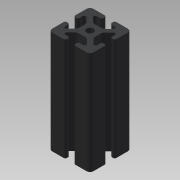
# Autodesk Inventor part: 40-4040-BLACK-FB
Saved by Autodesk Inventor 2013 (Build 170138000, 138)
## iProperties
Company: 80/20 Inc.
Created: 2014-04-23
Part Number: 40-4040-BLACK-FB
Material: Generic
Document SubType Name: Modeling
Designer: Ross Bowman
Density: 1 g/cm^3
Engineer: Ross Bowman
Catalog Web Link: 8020.net
Vendor: 80/20 Inc.
Material: 6105-T5 Aluminum
Author: Ross Bowman
Keywords: 80/20 , 8020 , T-Slot , Extrusion
Autodesk Inventor part; units mm, degrees
ref_plane "YZ Plane" through (0, 0, 0) normal (1, 0, 0) x (0, 1, 0)
ref_plane "XZ Plane" through (0, 0, 0) normal (0, 1, 0) x (-1, 0, 0)
ref_plane "XY Plane" through (0, 0, 0) normal (0, 0, 1) x (1, 0, 0)
sketch "Sketch1" plane through (0, 0, 0) normal (0, 0, 1) x (1, 0, 0)
  circle A0 centre (0, 0) radius 3.4
  arc A1 (-4.06, -17.0946) -> (-5.63, -15.5246) centre (-5.63, -17.0946) ccw
  line L0 (-5.63, -15.5246) -> (-8.715, -15.5246)
  arc A2 (-10.285, -13.9546) -> (-8.715, -15.5246) centre (-8.715, -13.9546) ccw
  line L1 (-10.285, -13.9546) -> (-10.285, -13.4925)
  arc A3 (-10.0624, -12.9551) -> (-10.285, -13.4925) centre (-9.525, -13.4925) ccw
  line L2 (-10.0624, -12.9551) -> (-6.2171, -9.1098)
  arc A4 (-2.7773, -7.685) -> (-6.2171, -9.1098) centre (-2.7773, -12.5496) ccw
  line L3 (-2.7773, -7.685) -> (2.7773, -7.685)
  arc A5 (6.2171, -9.1098) -> (2.7773, -7.685) centre (2.7773, -12.5496) ccw
  line L4 (6.2171, -9.1098) -> (10.0624, -12.9551)
  arc A6 (10.285, -13.4925) -> (10.0624, -12.9551) centre (9.525, -13.4925) ccw
  line L5 (10.285, -13.4925) -> (10.285, -13.9546)
  arc A7 (8.715, -15.5246) -> (10.285, -13.9546) centre (8.715, -13.9546) ccw
  line L6 (8.715, -15.5246) -> (5.63, -15.5246)
  arc A8 (5.63, -15.5246) -> (4.06, -17.0946) centre (5.63, -17.0946) ccw
  line L7 (4.06, -17.0946) -> (4.06, -18.43)
  arc A9 (4.06, -18.43) -> (5.63, -20) centre (5.63, -18.43) ccw
  line L8 (5.63, -20) -> (16.83, -20)
  arc A10 (16.83, -20) -> (20, -16.83) centre (16.83, -16.83) ccw
  line L9 (20, -16.83) -> (20, -5.63)
  arc A11 (20, -5.63) -> (18.43, -4.06) centre (18.43, -5.63) ccw
  line L10 (18.43, -4.06) -> (17.25, -4.06)
  arc A12 (17.25, -4.06) -> (15.68, -5.63) centre (17.25, -5.63) ccw
  line L11 (15.68, -5.63) -> (15.68, -8.7154)
  arc A13 (14.11, -10.2854) -> (15.68, -8.7154) centre (14.11, -8.7154) ccw
  line L12 (14.11, -10.2854) -> (13.6201, -10.2854)
  arc A14 (13.1637, -9.947) -> (13.6201, -10.2854) centre (13.8117, -9.55) ccw
  line L13 (13.1637, -9.947) -> (9.0762, -5.8595)
  arc A15 (7.685, -2.5008) -> (9.0762, -5.8595) centre (12.435, -2.5008) ccw
  line L14 (7.685, -2.5008) -> (7.685, 2.5008)
  arc A16 (9.0762, 5.8595) -> (7.685, 2.5008) centre (12.435, 2.5008) ccw
  line L15 (9.0762, 5.8595) -> (13.2795, 10.0628)
  arc A17 (13.8169, 10.2854) -> (13.2795, 10.0628) centre (13.8169, 9.5254) ccw
  line L16 (13.8169, 10.2854) -> (14.11, 10.2854)
  arc A18 (15.68, 8.7154) -> (14.11, 10.2854) centre (14.11, 8.7154) ccw
  line L17 (15.68, 8.7154) -> (15.68, 5.63)
  arc A19 (15.68, 5.63) -> (17.25, 4.06) centre (17.25, 5.63) ccw
  line L18 (17.25, 4.06) -> (18.43, 4.06)
  arc A20 (18.43, 4.06) -> (20, 5.63) centre (18.43, 5.63) ccw
  line L19 (20, 5.63) -> (20, 16.83)
  arc A21 (20, 16.83) -> (16.83, 20) centre (16.83, 16.83) ccw
  line L20 (16.83, 20) -> (5.63, 20)
  arc A22 (5.63, 20) -> (4.06, 18.43) centre (5.63, 18.43) ccw
  line L21 (4.06, 18.43) -> (4.06, 17.0946)
  arc A23 (4.06, 17.0946) -> (5.63, 15.5246) centre (5.63, 17.0946) ccw
  line L22 (5.63, 15.5246) -> (8.715, 15.5246)
  arc A24 (10.285, 13.9546) -> (8.715, 15.5246) centre (8.715, 13.9546) ccw
  line L23 (10.285, 13.9546) -> (10.285, 13.4925)
  arc A25 (10.0624, 12.9551) -> (10.285, 13.4925) centre (9.525, 13.4925) ccw
  line L24 (10.0624, 12.9551) -> (6.2171, 9.1098)
  arc A26 (2.7773, 7.685) -> (6.2171, 9.1098) centre (2.7773, 12.5496) ccw
  line L25 (2.7773, 7.685) -> (-2.7773, 7.685)
  arc A27 (-6.2171, 9.1098) -> (-2.7773, 7.685) centre (-2.7773, 12.5496) ccw
  line L26 (-6.2171, 9.1098) -> (-10.0624, 12.9551)
  arc A28 (-10.285, 13.4925) -> (-10.0624, 12.9551) centre (-9.525, 13.4925) ccw
  line L27 (-10.285, 13.4925) -> (-10.285, 13.9546)
  arc A29 (-8.715, 15.5246) -> (-10.285, 13.9546) centre (-8.715, 13.9546) ccw
  line L28 (-8.715, 15.5246) -> (-5.63, 15.5246)
  arc A30 (-5.63, 15.5246) -> (-4.06, 17.0946) centre (-5.63, 17.0946) ccw
  line L29 (-4.06, 17.0946) -> (-4.06, 18.43)
  arc A31 (-4.06, 18.43) -> (-5.63, 20) centre (-5.63, 18.43) ccw
  line L30 (-5.63, 20) -> (-16.83, 20)
  arc A32 (-16.83, 20) -> (-20, 16.83) centre (-16.83, 16.83) ccw
  line L31 (-20, 16.83) -> (-20, 5.573)
  arc A33 (-20, 5.573) -> (-18.43, 4.003) centre (-18.43, 5.573) ccw
  line L32 (-18.43, 4.003) -> (-17.25, 4.003)
  arc A34 (-17.25, 4.003) -> (-15.68, 5.573) centre (-17.25, 5.573) ccw
  line L33 (-15.68, 5.573) -> (-15.68, 8.4757)
  arc A35 (-14.0552, 10.0447) -> (-15.68, 8.4757) centre (-14.11, 8.4757) ccw
  line L34 (-14.0552, 10.0447) -> (-13.7199, 10.033)
  arc A36 (-13.0405, 9.8238) -> (-13.7199, 10.033) centre (-13.5779, 9.2864) ccw
  line L35 (-13.0405, 9.8238) -> (-9.0762, 5.8595)
  arc A37 (-7.685, 2.5008) -> (-9.0762, 5.8595) centre (-12.435, 2.5008) ccw
  line L36 (-7.685, 2.5008) -> (-7.685, -2.5008)
  arc A38 (-9.0762, -5.8595) -> (-7.685, -2.5008) centre (-12.435, -2.5008) ccw
  line L37 (-9.0762, -5.8595) -> (-13.2795, -10.0628)
  arc A39 (-13.8169, -10.2854) -> (-13.2795, -10.0628) centre (-13.8169, -9.5254) ccw
  line L38 (-13.8169, -10.2854) -> (-14.11, -10.2854)
  arc A40 (-15.68, -8.7154) -> (-14.11, -10.2854) centre (-14.11, -8.7154) ccw
  line L39 (-15.68, -8.7154) -> (-15.68, -5.7579)
  arc A41 (-15.68, -5.7579) -> (-17.25, -4.1204) centre (-17.2485, -5.6904) ccw
  line L40 (-17.25, -4.1204) -> (-18.43, -4.1204)
  arc A42 (-18.43, -4.1204) -> (-20, -5.7579) centre (-18.4315, -5.6904) ccw
  line L41 (-20, -5.7579) -> (-20, -17.0184)
  arc A43 (-20, -17.0184) -> (-16.6746, -20) centre (-16.8354, -16.8341) ccw
  line L42 (-16.6746, -20) -> (-5.63, -20)
  arc A44 (-5.63, -20) -> (-4.06, -18.43) centre (-5.63, -18.43) ccw
  line L43 (-4.06, -18.43) -> (-4.06, -17.0946)
  constraints: 88 end point, 88 point on circle, 45 centre point
extrude "Extrusion1" add sketch "Sketch1" against normal blind 100
body "Solid1"
